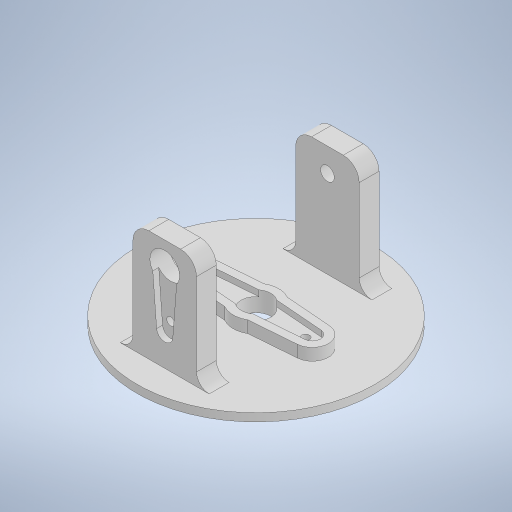
# Autodesk Inventor part: axis1
Saved by Autodesk Inventor 2023 (Build 270158000, 158)
## iProperties
Created: 2023-04-29
Part Number: axis1
Material: 一般
Document SubType Name: Modeling
Designer: taka2
Density: 1 g/cm^3
Appearance: 既定
Author: taka2
Autodesk Inventor part; units mm, degrees
ref_plane "YZ Plane" through (0, 0, 0) normal (1, 0, 0) x (0, 1, 0)
ref_plane "XZ Plane" through (0, 0, 0) normal (0, 1, 0) x (-1, 0, 0)
ref_plane "XY Plane" through (0, 0, 0) normal (0, 0, 1) x (1, 0, 0)
sketch "スケッチ1" plane through (0, 0, 0) normal (0, 1, 0) x (-1, 0, 0)
  circle A0 centre (0, 0) radius 30
  line L0 (0, -50.5872) -> (0, 52.7432)
  line L1 (-2.25, -3) -> (-14.3614, -2.0436)
  line L2 (47.5195, 0) -> (-63.2606, 0)
  line L3 (-2.25, 3) -> (-14.3614, 2.0436)
  arc A1 (-14.3614, 2.0436) -> (-14.3614, -2.0436) centre (-14.2, 0) ccw
  line L4 (2.25, -3) -> (14.3614, -2.0436)
  line L5 (2.25, 3) -> (14.3614, 2.0436)
  arc A2 (14.3614, -2.0436) -> (14.3614, 2.0436) centre (14.2, 0) ccw
  arc A3 (-2.25, -3) -> (2.25, -3) centre (0, 0) ccw
  arc A4 (2.25, 3) -> (-2.25, 3) centre (0, 0) ccw
  circle A5 centre (-12.5, 0) radius 1
  circle A6 centre (12.5, 0) radius 1
  line L6 (14.5188, -4.0374) -> (2.9201, -4.9533)
  arc A7 (-2.9201, -4.9533) -> (2.9201, -4.9533) centre (0, 0) ccw
  line L7 (-2.9201, -4.9533) -> (-14.5188, -4.0374)
  arc A8 (-14.5188, 4.0374) -> (-14.5188, -4.0374) centre (-14.2, 0) ccw
  line L8 (-14.5188, 4.0374) -> (-2.9201, 4.9533)
  arc A9 (2.9201, 4.9533) -> (-2.9201, 4.9533) centre (0, 0) ccw
  line L9 (2.9201, 4.9533) -> (14.5188, 4.0374)
  arc A10 (14.5188, -4.0374) -> (14.5188, 4.0374) centre (14.2, 0) ccw
  arc A11 (2.25, -3) -> (2.25, 3) centre (0, 0) ccw
  arc A12 (-2.25, 3) -> (-2.25, -3) centre (0, 0) ccw
  dimension "d0" = 60
  dimension "d1" = 14.2
  dimension "d2" = 2.05
  dimension "d3" = 6
  dimension "d5" = 12.5
  dimension "d6" = 2
  dimension "d7" = 2
  dimension "d10" = 3.75
  constraints: 21 point on circle, 20 end point, 13 centre point, 7 symmetric about line, 4 point on line, 2 coincident, 2 concentric, 1 horizontal, 1 tangent, 1 vertical, 11 other
  measures "d0" diameter of A0
  measures "d1" distance of A1.centre point (0, 0)
  measures "d2" radius of A1
  measures "d3" distance of L3.start L1.start
  measures "d5" distance of A5.centre point (0, 0)
  measures "d6" diameter of A5
  measures "d7" distance between parallel lines of L4 L6
  measures "d10" radius of A12
extrude "押し出し1" add sketch "スケッチ1" along normal blind 2 contours L2 A10 L9 A9 L0 A0 | A0 L0 A7 L6 A10 L2 | L0 A9 L8 A8 L2 A0 | A0 L2 A8 L7 A7 L0
extrude "押し出し2" add sketch "スケッチ1" along normal blind 5 contours A10 L6 A7 L0 A3 L4 A2 L2 | L2 A2 L5 A4 L0 A9 L9 A10 | L0 A4 L3 A1 L2 A8 L8 A9 | A7 L7 A8 L2 A1 L1 A3 L0
extrude "押し出し3" add sketch "スケッチ1" along normal blind 3.5 contours A2 L4 A11 L2 A6 | L2 A6 A11 L5 A2 | A1 L3 A12 L2 A5 | L2 A5 A12 L1 A1
sketch "スケッチ2" plane through (0, 2, 0) normal (0, 1, 0) x (1, 0, 0)
  line L0 (0, 57.7571) -> (0, -77.3728)
  line L1 (-74.0829, 0) -> (96.0409, 0)
  line L2 (-8, 18) -> (8, 18)
  line L3 (8, 18) -> (8, 23)
  line L4 (8, 23) -> (-8, 23)
  line L5 (-8, 23) -> (-8, 18)
  line L6 (-8, -18) -> (8, -18)
  line L7 (8, -18) -> (8, -23)
  line L8 (8, -23) -> (-8, -23)
  line L9 (-8, -23) -> (-8, -18)
  point P0 (0, 0)
  dimension "d15" = 36
  dimension "d16" = 16
  dimension "d17" = 5
  constraints: 20 end point, 4 symmetric about line, 2 horizontal, 2 parallel, 2 point on line, 1 perpendicular, 1 vertical, 1 other
  measures "d15" distance between parallel lines of L6 L2
  measures "d16" distance of L2.start L2.end
  measures "d17" distance of L2.end L3.end
extrude "押し出し4" add sketch "スケッチ2" along normal blind 28
sketch "スケッチ4" plane through (-8, 2, 23) normal (0, 0, 1) x (1, 0, 0)
  line L0 (0, 28) -> (16, 28) projected
  line L1 (8, 28) -> (8, 0)
  line L2 (38, 0) -> (-22, 0) projected
  circle A0 centre (8, 22) radius 3.75
  arc A1 (5.9564, 7.6386) -> (10.0436, 7.6386) centre (8, 7.8) ccw
  line L3 (5, 19.75) -> (5.9564, 7.6386)
  line L4 (11, 19.75) -> (10.0436, 7.6386)
  circle A2 centre (8, 9.5) radius 1
  point P0 (8, -2)
  dimension "d20" = 14.2
  dimension "d21" = 2
  dimension "d22" = 6
  dimension "d23" = 7.5
  dimension "d24" = 22
  dimension "d25" = 2.05
  dimension "d26" = 12.5
  constraints: 6 end point, 4 point on circle, 3 centre point, 3 point on line, 2 midpoint, 2 tangent, 1 other
  measures "d20" distance of A1.centre A0.centre
  measures "d21" diameter of A2
  measures "d22" distance of L3.start L4.start
  measures "d23" diameter of A0
  measures "d24" distance from line of L2 A0.centre
  measures "d25" radius of A1
  measures "d26" distance of A2.centre A0.centre
extrude "押し出し5" cut sketch "スケッチ4" against normal up to surface (5 mm away) contours A0 L1 | L1 A0 | A2 L1 | L1 A2
extrude "押し出し6" cut sketch "スケッチ4" against normal blind 1.5 contours A0 L4 A1 L1 A2 | L1 A2 A1 L3 A0
sketch "スケッチ5" plane through (8, 2, -23) normal (0, 0, -1) x (-1, 0, 0)
  line L0 (16, 28) -> (0, 28) projected
  line L1 (8, 28) -> (8, 0)
  line L2 (38, 0) -> (-22, 0) projected
  circle A0 centre (8, 22) radius 1.75
  circle A1 centre (8, 22) radius 3.75 projected
  point P0 (8, -2)
  dimension "d31" = 3.5
  constraints: 2 end point, 2 midpoint, 1 centre point, 1 concentric, 1 point on line
  measures "d31" diameter of A0
extrude "押し出し7" cut sketch "スケッチ5" against normal up to surface (5 mm away) contours A0 L1 | L1 A0
fillet "フィレット1" radius 3.2 4 edges at (8, 2, -20.5) (8, 2, 20.5) (-8, 2, -20.5) (-8, 2, 20.5)
fillet "フィレット2" radius 4 4 edges at (-8, 30, -20.5) (8, 30, -20.5) (-8, 30, 20.5) (8, 30, 20.5)
